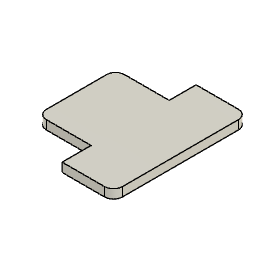
bottom_panel_opener (Autodesk Fusion 360 design; units mm, degrees)
Autodesk Fusion 360 part; units mm, degrees
sketch "Sketch1" plane through (0, 0, 0) normal (0, 0, 1) x (1, 0, 0)
  line L0 (-47.9346, 62.0575) -> (-70.9346, 62.0575)
  line L1 (-70.9346, 62.0575) -> (-70.9346, 122.0575)
  line L2 (-70.9346, 122.0575) -> (-47.9346, 122.0575)
  line L3 (-47.9346, 122.0575) -> (-47.9346, 62.0575)
  line L4 (-70.9346, 110) -> (-94.9346, 110)
  line L5 (-94.9346, 110) -> (-94.9346, 75)
  line L6 (-94.9346, 75) -> (-70.9346, 75)
  line L7 (-70.9346, 75) -> (-70.9346, 110)
  dimension "d1" = 35
  dimension "d3" = 60
  dimension "d4" = 24
  dimension "d10" = 23
  constraint horizontal L0
  constraint vertical L1
  constraint horizontal L2
  constraint vertical L3
  constraint horizontal L4
  constraint vertical L5
  constraint horizontal L6
  constraint vertical L7
  constraint coincident L1 L4.start
  measures "d1" distance of L4.end L5.end
  measures "d3" distance of L0.start L2.end
  measures "d4" distance of L4.start L4.end
  measures "d10" distance of L1 L3
extrude "Extrude1" add sketch "Sketch1" along normal blind 4
fillet "Fillet1" radius 4 2 edges at (-47.9346, 62.0575, 2) (-47.9346, 122.0575, 2)
fillet "Fillet1" radius 4 2 edges at (-94.9346, 75, 2) (-94.9346, 110, 2)
named bodies: "Bottom Panel Opener"
